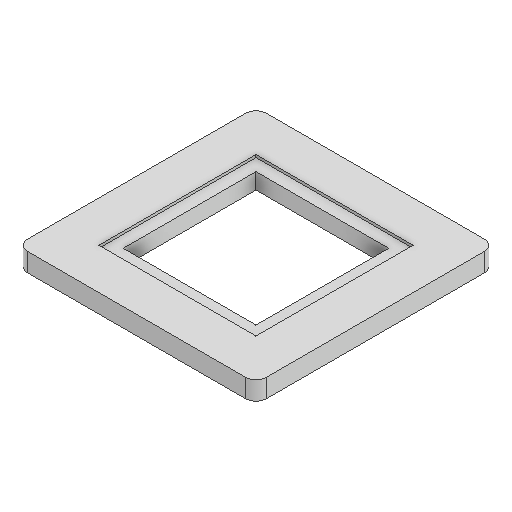
# Autodesk Inventor part: sup_soporte
Saved by Autodesk Inventor 2026.2 (Build 302298010, 298A)
## iProperties
Created: 2026-04-29
Part Number: sup_soporte
Material: Generic
Document SubType Name: Modeling
Designer: danie
Density: 1 g/cm^3
Appearance: Default
Author: danie
Autodesk Inventor part; units mm, degrees
ref_plane "YZ Plane" through (0, 0, 0) normal (1, 0, 0) x (0, 1, 0)
ref_plane "XZ Plane" through (0, 0, 0) normal (0, 1, 0) x (-1, 0, 0)
ref_plane "XY Plane" through (0, 0, 0) normal (0, 0, 1) x (1, 0, 0)
sketch "Sketch1" plane through (0, 0, 0) normal (0, 1, 0) x (-1, 0, 0)
  line L0 (-41, 45) -> (41, 45)
  line L1 (45, 41) -> (45, -41)
  line L2 (41, -45) -> (-41, -45)
  line L3 (-45, -41) -> (-45, 41)
  line L4 (-45, 45) -> (45, -45) construction
  line L5 (45, 45) -> (-45, -45) construction
  arc A0 (45, 41) -> (41, 45) centre (41, 41) ccw
  arc A1 (-41, 45) -> (-45, 41) centre (-41, 41) ccw
  arc A2 (-45, -41) -> (-41, -45) centre (-41, -41) ccw
  arc A3 (41, -45) -> (45, -41) centre (41, -41) ccw
  line L6 (25, 25) -> (-25, 25)
  line L7 (-25, 25) -> (-25, -25)
  line L8 (-25, -25) -> (25, -25)
  line L9 (25, -25) -> (25, 25)
  line L10 (25, 25) -> (-25, -25) construction
  line L11 (-25, 25) -> (25, -25) construction
  line L12 (29.575, 29.575) -> (-29.575, 29.575)
  line L13 (-29.575, 29.575) -> (-29.575, -29.575)
  line L14 (-29.575, -29.575) -> (29.575, -29.575)
  line L15 (29.575, -29.575) -> (29.575, 29.575)
  line L16 (29.575, 29.575) -> (-29.575, -29.575) construction
  line L17 (-29.575, 29.575) -> (29.575, -29.575) construction
  point P0 (0, 0)
  point P1 (0, -25)
  dimension "d0" = 90
  dimension "d1" = 90
  dimension "d2" = 4
  dimension "d3" = 50
  dimension "d4" = 50
  dimension "d5" = 59.15
  dimension "d6" = 59.15
  constraints: 36 end point, 10 point on line, 8 point on circle, 8 tangent, 7 midpoint, 6 parallel, 4 centre point, 3 equal radius, 3 horizontal, 3 perpendicular
  measures "d0" distance between parallel lines of L3 L1
  measures "d1" distance between parallel lines of L2 L0
  measures "d2" radius of A0
  measures "d3" distance from line of point (0, -25) L6
  measures "d4" distance between parallel lines of L7 L9
  measures "d5" distance between parallel lines of L14 L12
  measures "d6" distance between parallel lines of L13 L15
extrude "Extrusion1" add sketch "Sketch1" along normal blind 7 contours L0 A0 L1 A3 L2 A2 L3 A1
extrude "Extrusion2" add sketch "Sketch1" along normal blind 6 contours L15 L14 L13 L12
body "Solid1"
